Autodesk Fusion 360 part; units mm, degrees
(part 4 of 5)
sketch "Sketch5" plane through (0, 0, 10) normal (0, 0, 1) x (-1, 0, 0)
  arc A0 (206.7946, 25.828) -> (204.1076, 15.8) centre (264.6494, 4.9519) ccw
  arc A1 (201.8483, 14.174) -> (204.1076, 15.8) centre (202.1389, 16.1527) ccw
  line L0 (201.8483, 14.174) -> (193.8046, 15.3551)
  spline S0 degree 5 poles (193.8046, 15.3551) (193.7529, 15.3627) (193.6493, 15.3762) (193.4936, 15.3914) (193.2854, 15.4021) (193.0241, 15.4024) (192.7621, 15.3935) (192.4998, 15.379) (192.2373, 15.3616) (191.9747, 15.342) (191.712, 15.3201) (191.4492, 15.2951) (191.1864, 15.266) (190.9235, 15.2323) (190.6604, 15.1939) (190.3974, 15.1514) (190.1343, 15.1054) (189.8714, 15.0564) (189.6085, 15.0048) (189.3457, 14.9507) (189.083, 14.8941) (188.8205, 14.8347) (188.5581, 14.7725) (188.2959, 14.7074) (188.0338, 14.6394) (187.7718, 14.5688) (187.5101, 14.4956) (187.2485, 14.42) (186.9872, 14.342) (186.7261, 14.2617) (186.4653, 14.1791) (186.2047, 14.0941) (185.9443, 14.0069) (185.6842, 13.9173) (185.4244, 13.8255) (185.1649, 13.7314) (184.9057, 13.6352) (184.6467, 13.5369) (184.3881, 13.4364) (184.1298, 13.3338) (183.8719, 13.2292) (183.6143, 13.1226) (183.357, 13.0139) (183.1001, 12.9031) (182.8435, 12.7904) (182.5874, 12.6758) (182.3316, 12.5591) (182.0762, 12.4406) (181.8212, 12.3201) (181.5665, 12.1977) (181.3123, 12.0735) (181.0585, 11.9474) (180.8052, 11.8194) (180.5522, 11.6897) (180.2997, 11.5581) (180.0477, 11.4246) (179.7961, 11.2895) (179.5449, 11.1525) (179.2942, 11.0138) (179.044, 10.8733) (178.7943, 10.7311) (178.545, 10.5872) (178.2962, 10.4415) (178.048, 10.2942) (177.8002, 10.1451) (177.5529, 9.9945) (177.3062, 9.8421) (177.0599, 9.6881) (176.8142, 9.5325) (176.5691, 9.3752) (176.3244, 9.2163) (176.1291, 9.0879) (175.9829, 8.9909) (175.8855, 8.9259) (175.8369, 8.8933) knots 0 0 0 0 0 0 0.01428571 0.02857143 0.04285714 0.05714286 0.07142857 0.08571429 0.1 0.11428571 0.12857143 0.14285714 0.15714286 0.17142857 0.18571429 0.2 0.21428571 0.22857143 0.24285714 0.25714286 0.27142857 0.28571429 0.3 0.31428571 0.32857143 0.34285714 0.35714286 0.37142857 0.38571429 0.4 0.41428571 0.42857143 0.44285714 0.45714286 0.47142857 0.48571429 0.5 0.51428571 0.52857143 0.54285714 0.55714286 0.57142857 0.58571429 0.6 0.61428571 0.62857143 0.64285714 0.65714286 0.67142857 0.68571429 0.7 0.71428571 0.72857143 0.74285714 0.75714286 0.77142857 0.78571429 0.8 0.81428571 0.82857143 0.84285714 0.85714286 0.87142857 0.88571429 0.9 0.91428571 0.92857143 0.94285714 0.95714286 0.97142857 0.98571429 1 1 1 1 1 1
  arc A2 (175.8369, 8.8933) -> (175.8369, 1.0104) centre (264.6494, 4.9519) ccw
  spline S1 degree 5 poles (175.8369, 1.0104) (175.8855, 0.9779) (175.9829, 0.9129) (176.1291, 0.8158) (176.3244, 0.6874) (176.5691, 0.5285) (176.8142, 0.3713) (177.0599, 0.2156) (177.3062, 0.0616) (177.5529, -0.0907) (177.8002, -0.2414) (178.048, -0.3905) (178.2962, -0.5378) (178.545, -0.6834) (178.7943, -0.8274) (179.044, -0.9696) (179.2942, -1.11) (179.5449, -1.2488) (179.7961, -1.3857) (180.0477, -1.5209) (180.2997, -1.6543) (180.5522, -1.7859) (180.8052, -1.9157) (181.0585, -2.0437) (181.3123, -2.1698) (181.5665, -2.294) (181.8212, -2.4164) (182.0762, -2.5368) (182.3316, -2.6554) (182.5874, -2.772) (182.8435, -2.8867) (183.1001, -2.9994) (183.357, -3.1101) (183.6143, -3.2188) (183.8719, -3.3255) (184.1298, -3.4301) (184.3881, -3.5327) (184.6467, -3.6331) (184.9057, -3.7315) (185.1649, -3.8277) (185.4244, -3.9218) (185.6842, -4.0136) (185.9443, -4.1031) (186.2047, -4.1904) (186.4653, -4.2753) (186.7261, -4.358) (186.9872, -4.4383) (187.2485, -4.5163) (187.5101, -4.5919) (187.7718, -4.6651) (188.0338, -4.7357) (188.2959, -4.8036) (188.5581, -4.8688) (188.8205, -4.931) (189.083, -4.9903) (189.3457, -5.047) (189.6085, -5.1011) (189.8714, -5.1527) (190.1343, -5.2017) (190.3974, -5.2477) (190.6604, -5.2902) (190.9235, -5.3286) (191.1864, -5.3623) (191.4492, -5.3914) (191.712, -5.4164) (191.9747, -5.4383) (192.2373, -5.4578) (192.4998, -5.4753) (192.7621, -5.4898) (193.0241, -5.4987) (193.2854, -5.4984) (193.4936, -5.4877) (193.6493, -5.4725) (193.7529, -5.459) (193.8046, -5.4514) knots -1 -1 -1 -1 -1 -1 -0.98571429 -0.97142857 -0.95714286 -0.94285714 -0.92857143 -0.91428571 -0.9 -0.88571429 -0.87142857 -0.85714286 -0.84285714 -0.82857143 -0.81428571 -0.8 -0.78571429 -0.77142857 -0.75714286 -0.74285714 -0.72857143 -0.71428571 -0.7 -0.68571429 -0.67142857 -0.65714286 -0.64285714 -0.62857143 -0.61428571 -0.6 -0.58571429 -0.57142857 -0.55714286 -0.54285714 -0.52857143 -0.51428571 -0.5 -0.48571429 -0.47142857 -0.45714286 -0.44285714 -0.42857143 -0.41428571 -0.4 -0.38571429 -0.37142857 -0.35714286 -0.34285714 -0.32857143 -0.31428571 -0.3 -0.28571429 -0.27142857 -0.25714286 -0.24285714 -0.22857143 -0.21428571 -0.2 -0.18571429 -0.17142857 -0.15714286 -0.14285714 -0.12857143 -0.11428571 -0.1 -0.08571429 -0.07142857 -0.05714286 -0.04285714 -0.02857143 -0.01428571 0 0 0 0 0 0
  line L1 (193.8046, -5.4514) -> (201.8483, -4.2702)
  arc A3 (204.1076, -5.8963) -> (201.8483, -4.2702) centre (202.1389, -6.249) ccw
  arc A4 (204.1076, -5.8963) -> (206.7946, -15.9243) centre (264.6494, 4.9519) ccw
  arc A5 (205.651, -18.4621) -> (206.7946, -15.9243) centre (204.9133, -16.6032) ccw
  line L2 (205.651, -18.4621) -> (198.0944, -21.461)
  spline S2 degree 5 poles (198.0944, -21.461) (198.0458, -21.4803) (197.9494, -21.5204) (197.8069, -21.5851) (197.6212, -21.68) (197.3948, -21.8104) (197.1724, -21.9491) (196.9524, -22.0928) (196.7338, -22.2391) (196.5162, -22.3874) (196.2996, -22.5377) (196.0846, -22.6907) (195.8715, -22.8473) (195.6607, -23.008) (195.452, -23.1727) (195.2455, -23.3411) (195.0407, -23.5125) (194.8375, -23.6864) (194.6356, -23.8625) (194.4351, -24.0407) (194.2359, -24.2211) (194.0383, -24.4038) (193.8421, -24.5889) (193.6475, -24.7764) (193.4545, -24.9663) (193.263, -25.1584) (193.0729, -25.3527) (192.8842, -25.549) (192.6969, -25.7472) (192.511, -25.9473) (192.3264, -26.1492) (192.1431, -26.3531) (191.9613, -26.5588) (191.7808, -26.7664) (191.6017, -26.9759) (191.424, -27.1871) (191.2476, -27.4) (191.0726, -27.6147) (190.8988, -27.831) (190.7264, -28.0489) (190.5553, -28.2685) (190.3856, -28.4897) (190.2171, -28.7125) (190.05, -28.9368) (189.8842, -29.1627) (189.7197, -29.3901) (189.5564, -29.619) (189.3945, -29.8494) (189.2339, -30.0812) (189.0746, -30.3145) (188.9166, -30.5492) (188.7598, -30.7853) (188.6044, -31.0228) (188.4502, -31.2616) (188.2974, -31.5019) (188.1458, -31.7434) (187.9955, -31.9863) (187.8465, -32.2305) (187.6987, -32.476) (187.5523, -32.7227) (187.4071, -32.9708) (187.2632, -33.22) (187.1206, -33.4706) (186.9792, -33.7223) (186.8391, -33.9752) (186.7003, -34.2294) (186.5628, -34.4847) (186.4266, -34.7412) (186.2916, -34.9988) (186.1579, -35.2576) (186.0255, -35.5175) (185.9206, -35.7264) (185.8425, -35.8835) (185.7906, -35.9885) (185.7648, -36.0411) knots 0 0 0 0 0 0 0.01428571 0.02857143 0.04285714 0.05714286 0.07142857 0.08571429 0.1 0.11428571 0.12857143 0.14285714 0.15714286 0.17142857 0.18571429 0.2 0.21428571 0.22857143 0.24285714 0.25714286 0.27142857 0.28571429 0.3 0.31428571 0.32857143 0.34285714 0.35714286 0.37142857 0.38571429 0.4 0.41428571 0.42857143 0.44285714 0.45714286 0.47142857 0.48571429 0.5 0.51428571 0.52857143 0.54285714 0.55714286 0.57142857 0.58571429 0.6 0.61428571 0.62857143 0.64285714 0.65714286 0.67142857 0.68571429 0.7 0.71428571 0.72857143 0.74285714 0.75714286 0.77142857 0.78571429 0.8 0.81428571 0.82857143 0.84285714 0.85714286 0.87142857 0.88571429 0.9 0.91428571 0.92857143 0.94285714 0.95714286 0.97142857 0.98571429 1 1 1 1 1 1
  arc A6 (185.7648, -36.0411) -> (189.7062, -42.8678) centre (264.6494, 4.9519) ccw
  spline S3 degree 5 poles (189.7062, -42.8678) (189.7646, -42.8717) (189.8815, -42.8793) (190.0566, -42.8902) (190.2899, -42.9038) (190.5813, -42.9191) (190.8722, -42.9327) (191.1628, -42.9446) (191.4531, -42.9548) (191.7429, -42.9634) (192.0324, -42.9703) (192.3215, -42.9755) (192.6102, -42.9789) (192.8985, -42.9807) (193.1863, -42.9807) (193.4737, -42.979) (193.7606, -42.9755) (194.0471, -42.9703) (194.3331, -42.9633) (194.6186, -42.9546) (194.9035, -42.9441) (195.188, -42.9318) (195.472, -42.9178) (195.7554, -42.9019) (196.0382, -42.8842) (196.3205, -42.8647) (196.6022, -42.8434) (196.8832, -42.8202) (197.1637, -42.7952) (197.4436, -42.7683) (197.7227, -42.7395) (198.0013, -42.7088) (198.2791, -42.6763) (198.5563, -42.6418) (198.8327, -42.6053) (199.1084, -42.5669) (199.3834, -42.5266) (199.6576, -42.4843) (199.931, -42.44) (200.2036, -42.3938) (200.4754, -42.3454) (200.7463, -42.2951) (201.0163, -42.2426) (201.2854, -42.188) (201.5536, -42.1312) (201.8208, -42.0723) (202.087, -42.0113) (202.3523, -41.9482) (202.6167, -41.8829) (202.8799, -41.8155) (203.1421, -41.7457) (203.4031, -41.6734) (203.6627, -41.5987) (203.9211, -41.5214) (204.1781, -41.4415) (204.4339, -41.3593) (204.6885, -41.2747) (204.942, -41.188) (205.1942, -41.0989) (205.4451, -41.0073) (205.6941, -40.9125) (205.9411, -40.8142) (206.1857, -40.712) (206.4278, -40.6058) (206.6679, -40.4961) (206.9063, -40.3837) (207.1435, -40.2693) (207.3796, -40.1531) (207.614, -40.0345) (207.8453, -39.9113) (208.0715, -39.7804) (208.2465, -39.667) (208.3737, -39.576) (208.4567, -39.5125) (208.4977, -39.4801) knots -1 -1 -1 -1 -1 -1 -0.98571429 -0.97142857 -0.95714286 -0.94285714 -0.92857143 -0.91428571 -0.9 -0.88571429 -0.87142857 -0.85714286 -0.84285714 -0.82857143 -0.81428571 -0.8 -0.78571429 -0.77142857 -0.75714286 -0.74285714 -0.72857143 -0.71428571 -0.7 -0.68571429 -0.67142857 -0.65714286 -0.64285714 -0.62857143 -0.61428571 -0.6 -0.58571429 -0.57142857 -0.55714286 -0.54285714 -0.52857143 -0.51428571 -0.5 -0.48571429 -0.47142857 -0.45714286 -0.44285714 -0.42857143 -0.41428571 -0.4 -0.38571429 -0.37142857 -0.35714286 -0.34285714 -0.32857143 -0.31428571 -0.3 -0.28571429 -0.27142857 -0.25714286 -0.24285714 -0.22857143 -0.21428571 -0.2 -0.18571429 -0.17142857 -0.15714286 -0.14285714 -0.12857143 -0.11428571 -0.1 -0.08571429 -0.07142857 -0.05714286 -0.04285714 -0.02857143 -0.01428571 0 0 0 0 0 0
  line L3 (208.4977, -39.4801) -> (214.8731, -34.4353)
  arc A7 (217.6427, -34.7138) -> (214.8731, -34.4353) centre (216.1142, -36.0036) ccw
  arc A8 (217.6427, -34.7138) -> (224.9837, -42.0549) centre (264.6494, 4.9519) ccw
  arc A9 (225.2623, -44.8244) -> (224.9837, -42.0549) centre (223.6939, -43.5834) ccw
  line L4 (225.2623, -44.8244) -> (220.2175, -51.1999)
  spline S4 degree 5 poles (220.2175, -51.1999) (220.1851, -51.2409) (220.1216, -51.3238) (220.0306, -51.4511) (219.9172, -51.6261) (219.7863, -51.8522) (219.6631, -52.0835) (219.5444, -52.318) (219.4283, -52.554) (219.3139, -52.7913) (219.2015, -53.0297) (219.0918, -53.2697) (218.9856, -53.5119) (218.8833, -53.7565) (218.785, -54.0035) (218.6903, -54.2525) (218.5987, -54.5033) (218.5096, -54.7556) (218.4228, -55.009) (218.3383, -55.2637) (218.256, -55.5195) (218.1762, -55.7765) (218.0989, -56.0348) (218.0241, -56.2945) (217.9519, -56.5555) (217.8821, -56.8176) (217.8146, -57.0809) (217.7494, -57.3452) (217.6862, -57.6105) (217.6252, -57.8768) (217.5664, -58.144) (217.5096, -58.4122) (217.455, -58.6813) (217.4025, -58.9513) (217.3521, -59.2222) (217.3038, -59.494) (217.2575, -59.7666) (217.2133, -60.04) (217.171, -60.3142) (217.1306, -60.5892) (217.0923, -60.8649) (217.0558, -61.1413) (217.0213, -61.4184) (216.9887, -61.6963) (216.9581, -61.9748) (216.9293, -62.254) (216.9024, -62.5339) (216.8774, -62.8143) (216.8542, -63.0954) (216.8329, -63.3771) (216.8134, -63.6594) (216.7957, -63.9422) (216.7798, -64.2256) (216.7657, -64.5096) (216.7535, -64.794) (216.743, -65.079) (216.7342, -65.3645) (216.7273, -65.6505) (216.7221, -65.937) (216.7186, -66.2239) (216.7169, -66.5113) (216.7169, -66.7991) (216.7187, -67.0874) (216.7221, -67.3761) (216.7273, -67.6652) (216.7342, -67.9546) (216.7427, -68.2445) (216.753, -68.5348) (216.7649, -68.8254) (216.7785, -69.1163) (216.7938, -69.4076) (216.8074, -69.641) (216.8183, -69.8161) (216.8259, -69.933) (216.8298, -69.9914) knots 0 0 0 0 0 0 0.01428571 0.02857143 0.04285714 0.05714286 0.07142857 0.08571429 0.1 0.11428571 0.12857143 0.14285714 0.15714286 0.17142857 0.18571429 0.2 0.21428571 0.22857143 0.24285714 0.25714286 0.27142857 0.28571429 0.3 0.31428571 0.32857143 0.34285714 0.35714286 0.37142857 0.38571429 0.4 0.41428571 0.42857143 0.44285714 0.45714286 0.47142857 0.48571429 0.5 0.51428571 0.52857143 0.54285714 0.55714286 0.57142857 0.58571429 0.6 0.61428571 0.62857143 0.64285714 0.65714286 0.67142857 0.68571429 0.7 0.71428571 0.72857143 0.74285714 0.75714286 0.77142857 0.78571429 0.8 0.81428571 0.82857143 0.84285714 0.85714286 0.87142857 0.88571429 0.9 0.91428571 0.92857143 0.94285714 0.95714286 0.97142857 0.98571429 1 1 1 1 1 1
  arc A10 (216.8298, -69.9914) -> (223.6565, -73.9328) centre (264.6494, 4.9519) ccw
  spline S5 degree 5 poles (223.6565, -73.9328) (223.7091, -73.9069) (223.814, -73.8551) (223.9712, -73.777) (224.18, -73.6721) (224.44, -73.5397) (224.6987, -73.406) (224.9564, -73.271) (225.2129, -73.1348) (225.4682, -72.9972) (225.7223, -72.8584) (225.9753, -72.7184) (226.227, -72.577) (226.4775, -72.4344) (226.7268, -72.2905) (226.9748, -72.1453) (227.2216, -71.9989) (227.4671, -71.8511) (227.7113, -71.7021) (227.9542, -71.5518) (228.1957, -71.4002) (228.4359, -71.2473) (228.6748, -71.0932) (228.9123, -70.9377) (229.1484, -70.781) (229.3831, -70.623) (229.6164, -70.4637) (229.8482, -70.303) (230.0786, -70.1411) (230.3075, -69.9779) (230.5349, -69.8134) (230.7608, -69.6476) (230.9851, -69.4804) (231.2079, -69.312) (231.4291, -69.1422) (231.6486, -68.9711) (231.8666, -68.7987) (232.0829, -68.625) (232.2976, -68.45) (232.5105, -68.2736) (232.7217, -68.0958) (232.9311, -67.9167) (233.1387, -67.7363) (233.3445, -67.5544) (233.5483, -67.3712) (233.7503, -67.1866) (233.9504, -67.0007) (234.1486, -66.8133) (234.3449, -66.6247) (234.5391, -66.4346) (234.7313, -66.2431) (234.9212, -66.05) (235.1087, -65.8555) (235.2938, -65.6593) (235.4764, -65.4617) (235.6568, -65.2625) (235.8351, -65.062) (236.0112, -64.8601) (236.1851, -64.6569) (236.3565, -64.4521) (236.5248, -64.2455) (236.6895, -64.0369) (236.8503, -63.8261) (237.0069, -63.613) (237.1599, -63.398) (237.3102, -63.1814) (237.4584, -62.9638) (237.6048, -62.7451) (237.7485, -62.5252) (237.8872, -62.3028) (238.0176, -62.0764) (238.1125, -61.8907) (238.1772, -61.7482) (238.2173, -61.6518) (238.2365, -61.6032) knots -1 -1 -1 -1 -1 -1 -0.98571429 -0.97142857 -0.95714286 -0.94285714 -0.92857143 -0.91428571 -0.9 -0.88571429 -0.87142857 -0.85714286 -0.84285714 -0.82857143 -0.81428571 -0.8 -0.78571429 -0.77142857 -0.75714286 -0.74285714 -0.72857143 -0.71428571 -0.7 -0.68571429 -0.67142857 -0.65714286 -0.64285714 -0.62857143 -0.61428571 -0.6 -0.58571429 -0.57142857 -0.55714286 -0.54285714 -0.52857143 -0.51428571 -0.5 -0.48571429 -0.47142857 -0.45714286 -0.44285714 -0.42857143 -0.41428571 -0.4 -0.38571429 -0.37142857 -0.35714286 -0.34285714 -0.32857143 -0.31428571 -0.3 -0.28571429 -0.27142857 -0.25714286 -0.24285714 -0.22857143 -0.21428571 -0.2 -0.18571429 -0.17142857 -0.15714286 -0.14285714 -0.12857143 -0.11428571 -0.1 -0.08571429 -0.07142857 -0.05714286 -0.04285714 -0.02857143 -0.01428571 0 0 0 0 0 0
  line L5 (238.2365, -61.6032) -> (241.2355, -54.0465)
  arc A11 (243.7733, -52.903) -> (241.2355, -54.0465) centre (243.0944, -54.7843) ccw
  arc A12 (243.7733, -52.903) -> (253.8013, -55.59) centre (264.6494, 4.9519) ccw
  arc A13 (255.4273, -57.8492) -> (253.8013, -55.59) centre (253.4486, -57.5587) ccw
  line L6 (255.4273, -57.8492) -> (254.2461, -65.8929)
  spline S6 degree 5 poles (254.2461, -65.8929) (254.2386, -65.9447) (254.225, -66.0482) (254.2099, -66.2039) (254.1992, -66.4122) (254.1989, -66.6735) (254.2078, -66.9354) (254.2223, -67.1978) (254.2397, -67.4603) (254.2593, -67.7229) (254.2812, -67.9856) (254.3062, -68.2483) (254.3353, -68.5112) (254.369, -68.7741) (254.4074, -69.0371) (254.4499, -69.3002) (254.4959, -69.5632) (254.5449, -69.8262) (254.5965, -70.0891) (254.6506, -70.3519) (254.7072, -70.6145) (254.7666, -70.8771) (254.8288, -71.1395) (254.8939, -71.4017) (254.9619, -71.6638) (255.0325, -71.9258) (255.1057, -72.1875) (255.1813, -72.449) (255.2593, -72.7104) (255.3396, -72.9715) (255.4222, -73.2323) (255.5072, -73.4929) (255.5944, -73.7533) (255.684, -74.0134) (255.7758, -74.2732) (255.8699, -74.5327) (255.9661, -74.7919) (256.0644, -75.0508) (256.1649, -75.3095) (256.2675, -75.5677) (256.3721, -75.8257) (256.4787, -76.0833) (256.5874, -76.3406) (256.6981, -76.5975) (256.8109, -76.854) (256.9255, -77.1102) (257.0422, -77.366) (257.1607, -77.6214) (257.2812, -77.8764) (257.4036, -78.131) (257.5278, -78.3852) (257.6539, -78.639) (257.7819, -78.8924) (257.9116, -79.1453) (258.0432, -79.3978) (258.1766, -79.6499) (258.3118, -79.9015) (258.4488, -80.1527) (258.5875, -80.4033) (258.728, -80.6536) (258.8702, -80.9033) (259.0141, -81.1526) (259.1598, -81.4013) (259.3071, -81.6496) (259.4561, -81.8974) (259.6068, -82.1447) (259.7592, -82.3914) (259.9132, -82.6376) (260.0688, -82.8834) (260.2261, -83.1285) (260.385, -83.3732) (260.5134, -83.5685) (260.6104, -83.7147) (260.6754, -83.8121) (260.708, -83.8607) knots 0 0 0 0 0 0 0.01428571 0.02857143 0.04285714 0.05714286 0.07142857 0.08571429 0.1 0.11428571 0.12857143 0.14285714 0.15714286 0.17142857 0.18571429 0.2 0.21428571 0.22857143 0.24285714 0.25714286 0.27142857 0.28571429 0.3 0.31428571 0.32857143 0.34285714 0.35714286 0.37142857 0.38571429 0.4 0.41428571 0.42857143 0.44285714 0.45714286 0.47142857 0.48571429 0.5 0.51428571 0.52857143 0.54285714 0.55714286 0.57142857 0.58571429 0.6 0.61428571 0.62857143 0.64285714 0.65714286 0.67142857 0.68571429 0.7 0.71428571 0.72857143 0.74285714 0.75714286 0.77142857 0.78571429 0.8 0.81428571 0.82857143 0.84285714 0.85714286 0.87142857 0.88571429 0.9 0.91428571 0.92857143 0.94285714 0.95714286 0.97142857 0.98571429 1 1 1 1 1 1
  arc A14 (260.708, -83.8607) -> (268.5908, -83.8607) centre (264.6494, 4.9519) ccw
  spline S7 degree 5 poles (268.5908, -83.8607) (268.6234, -83.8121) (268.6884, -83.7147) (268.7855, -83.5685) (268.9139, -83.3732) (269.0728, -83.1285) (269.23, -82.8834) (269.3857, -82.6376) (269.5397, -82.3914) (269.692, -82.1447) (269.8427, -81.8974) (269.9917, -81.6496) (270.1391, -81.4013) (270.2847, -81.1526) (270.4287, -80.9033) (270.5709, -80.6536) (270.7113, -80.4033) (270.8501, -80.1527) (270.987, -79.9015) (271.1222, -79.6499) (271.2556, -79.3978) (271.3872, -79.1453) (271.517, -78.8924) (271.645, -78.639) (271.7711, -78.3852) (271.8953, -78.131) (272.0177, -77.8764) (272.1381, -77.6214) (272.2567, -77.366) (272.3733, -77.1102) (272.488, -76.854) (272.6007, -76.5975) (272.7114, -76.3406) (272.8201, -76.0833) (272.9268, -75.8257) (273.0314, -75.5677) (273.134, -75.3095) (273.2344, -75.0508) (273.3328, -74.7919) (273.429, -74.5327) (273.5231, -74.2732) (273.6149, -74.0134) (273.7044, -73.7533) (273.7917, -73.4929) (273.8766, -73.2323) (273.9592, -72.9715) (274.0396, -72.7104) (274.1175, -72.449) (274.1932, -72.1875) (274.2664, -71.9258) (274.337, -71.6638) (274.4049, -71.4017) (274.47, -71.1395) (274.5323, -70.8771) (274.5916, -70.6145) (274.6483, -70.3519) (274.7024, -70.0891) (274.754, -69.8262) (274.803, -69.5632) (274.849, -69.3002) (274.8915, -69.0371) (274.9299, -68.7741) (274.9636, -68.5112) (274.9927, -68.2483) (275.0177, -67.9856) (275.0396, -67.7229) (275.0591, -67.4603) (275.0766, -67.1978) (275.0911, -66.9354) (275.1, -66.6735) (275.0997, -66.4122) (275.089, -66.2039) (275.0738, -66.0482) (275.0603, -65.9447) (275.0527, -65.8929) knots -1 -1 -1 -1 -1 -1 -0.98571429 -0.97142857 -0.95714286 -0.94285714 -0.92857143 -0.91428571 -0.9 -0.88571429 -0.87142857 -0.85714286 -0.84285714 -0.82857143 -0.81428571 -0.8 -0.78571429 -0.77142857 -0.75714286 -0.74285714 -0.72857143 -0.71428571 -0.7 -0.68571429 -0.67142857 -0.65714286 -0.64285714 -0.62857143 -0.61428571 -0.6 -0.58571429 -0.57142857 -0.55714286 -0.54285714 -0.52857143 -0.51428571 -0.5 -0.48571429 -0.47142857 -0.45714286 -0.44285714 -0.42857143 -0.41428571 -0.4 -0.38571429 -0.37142857 -0.35714286 -0.34285714 -0.32857143 -0.31428571 -0.3 -0.28571429 -0.27142857 -0.25714286 -0.24285714 -0.22857143 -0.21428571 -0.2 -0.18571429 -0.17142857 -0.15714286 -0.14285714 -0.12857143 -0.11428571 -0.1 -0.08571429 -0.07142857 -0.05714286 -0.04285714 -0.02857143 -0.01428571 0 0 0 0 0 0
  line L7 (275.0527, -65.8929) -> (273.8715, -57.8492)
  arc A15 (275.4976, -55.59) -> (273.8715, -57.8492) centre (275.8503, -57.5587) ccw
  arc A16 (275.4976, -55.59) -> (285.5256, -52.903) centre (264.6494, 4.9519) ccw
  arc A17 (288.0634, -54.0465) -> (285.5256, -52.903) centre (286.2045, -54.7843) ccw
  line L8 (288.0634, -54.0465) -> (291.0623, -61.6032)
  spline S8 degree 5 poles (291.0623, -61.6032) (291.0816, -61.6518) (291.1217, -61.7482) (291.1864, -61.8907) (291.2813, -62.0764) (291.4117, -62.3028) (291.5503, -62.5252) (291.6941, -62.7451) (291.8404, -62.9638) (291.9887, -63.1814) (292.139, -63.398) (292.292, -63.613) (292.4486, -63.8261) (292.6093, -64.0369) (292.774, -64.2455) (292.9424, -64.4521) (293.1138, -64.6569) (293.2877, -64.8601) (293.4638, -65.062) (293.642, -65.2625) (293.8224, -65.4617) (294.0051, -65.6593) (294.1902, -65.8555) (294.3777, -66.05) (294.5676, -66.2431) (294.7597, -66.4346) (294.954, -66.6247) (295.1503, -66.8133) (295.3485, -67.0007) (295.5486, -67.1866) (295.7505, -67.3712) (295.9544, -67.5544) (296.1601, -67.7363) (296.3677, -67.9167) (296.5772, -68.0958) (296.7884, -68.2736) (297.0013, -68.45) (297.216, -68.625) (297.4323, -68.7987) (297.6502, -68.9711) (297.8698, -69.1422) (298.091, -69.312) (298.3138, -69.4804) (298.5381, -69.6476) (298.764, -69.8134) (298.9914, -69.9779) (299.2203, -70.1411) (299.4507, -70.303) (299.6825, -70.4637) (299.9158, -70.623) (300.1505, -70.781) (300.3866, -70.9377) (300.6241, -71.0932) (300.8629, -71.2473) (301.1032, -71.4002) (301.3447, -71.5518) (301.5876, -71.7021) (301.8318, -71.8511) (302.0773, -71.9989) (302.324, -72.1453) (302.5721, -72.2905) (302.8213, -72.4344) (303.0719, -72.577) (303.3236, -72.7184) (303.5765, -72.8584) (303.8307, -72.9972) (304.086, -73.1348) (304.3425, -73.271) (304.6001, -73.406) (304.8589, -73.5397) (305.1188, -73.6721) (305.3277, -73.777) (305.4848, -73.8551) (305.5898, -73.9069) (305.6424, -73.9328) knots 0 0 0 0 0 0 0.01428571 0.02857143 0.04285714 0.05714286 0.07142857 0.08571429 0.1 0.11428571 0.12857143 0.14285714 0.15714286 0.17142857 0.18571429 0.2 0.21428571 0.22857143 0.24285714 0.25714286 0.27142857 0.28571429 0.3 0.31428571 0.32857143 0.34285714 0.35714286 0.37142857 0.38571429 0.4 0.41428571 0.42857143 0.44285714 0.45714286 0.47142857 0.48571429 0.5 0.51428571 0.52857143 0.54285714 0.55714286 0.57142857 0.58571429 0.6 0.61428571 0.62857143 0.64285714 0.65714286 0.67142857 0.68571429 0.7 0.71428571 0.72857143 0.74285714 0.75714286 0.77142857 0.78571429 0.8 0.81428571 0.82857143 0.84285714 0.85714286 0.87142857 0.88571429 0.9 0.91428571 0.92857143 0.94285714 0.95714286 0.97142857 0.98571429 1 1 1 1 1 1
  arc A18 (305.6424, -73.9328) -> (312.4691, -69.9914) centre (264.6494, 4.9519) ccw
  spline S9 degree 5 poles (312.4691, -69.9914) (312.473, -69.933) (312.4806, -69.8161) (312.4915, -69.641) (312.5051, -69.4076) (312.5203, -69.1163) (312.534, -68.8254) (312.5459, -68.5348) (312.5561, -68.2445) (312.5647, -67.9546) (312.5716, -67.6652) (312.5768, -67.3761) (312.5802, -67.0874) (312.582, -66.7991) (312.582, -66.5113) (312.5803, -66.2239) (312.5768, -65.937) (312.5716, -65.6505) (312.5646, -65.3645) (312.5559, -65.079) (312.5454, -64.794) (312.5331, -64.5096) (312.5191, -64.2256) (312.5032, -63.9422) (312.4855, -63.6594) (312.466, -63.3771) (312.4447, -63.0954) (312.4215, -62.8143) (312.3965, -62.5339) (312.3696, -62.254) (312.3408, -61.9748) (312.3101, -61.6963) (312.2775, -61.4184) (312.243, -61.1413) (312.2066, -60.8649) (312.1682, -60.5892) (312.1279, -60.3142) (312.0856, -60.04) (312.0413, -59.7666) (311.9951, -59.494) (311.9467, -59.2222) (311.8964, -58.9513) (311.8439, -58.6813) (311.7893, -58.4122) (311.7325, -58.144) (311.6736, -57.8768) (311.6126, -57.6105) (311.5495, -57.3452) (311.4842, -57.0809) (311.4168, -56.8176) (311.347, -56.5555) (311.2747, -56.2945) (311.2, -56.0348) (311.1227, -55.7765) (311.0428, -55.5195) (310.9606, -55.2637) (310.876, -55.009) (310.7893, -54.7556) (310.7002, -54.5033) (310.6086, -54.2525) (310.5138, -54.0035) (310.4155, -53.7565) (310.3133, -53.5119) (310.2071, -53.2697) (310.0974, -53.0297) (309.985, -52.7913) (309.8706, -52.554) (309.7544, -52.318) (309.6358, -52.0835) (309.5126, -51.8522) (309.3817, -51.6261) (309.2683, -51.4511) (309.1773, -51.3238) (309.1138, -51.2409) (309.0814, -51.1999) knots -1 -1 -1 -1 -1 -1 -0.98571429 -0.97142857 -0.95714286 -0.94285714 -0.92857143 -0.91428571 -0.9 -0.88571429 -0.87142857 -0.85714286 -0.84285714 -0.82857143 -0.81428571 -0.8 -0.78571429 -0.77142857 -0.75714286 -0.74285714 -0.72857143 -0.71428571 -0.7 -0.68571429 -0.67142857 -0.65714286 -0.64285714 -0.62857143 -0.61428571 -0.6 -0.58571429 -0.57142857 -0.55714286 -0.54285714 -0.52857143 -0.51428571 -0.5 -0.48571429 -0.47142857 -0.45714286 -0.44285714 -0.42857143 -0.41428571 -0.4 -0.38571429 -0.37142857 -0.35714286 -0.34285714 -0.32857143 -0.31428571 -0.3 -0.28571429 -0.27142857 -0.25714286 -0.24285714 -0.22857143 -0.21428571 -0.2 -0.18571429 -0.17142857 -0.15714286 -0.14285714 -0.12857143 -0.11428571 -0.1 -0.08571429 -0.07142857 -0.05714286 -0.04285714 -0.02857143 -0.01428571 0 0 0 0 0 0
  line L9 (309.0814, -51.1999) -> (304.0366, -44.8244)
  arc A19 (304.3151, -42.0549) -> (304.0366, -44.8244) centre (305.6049, -43.5834) ccw
  arc A20 (304.3151, -42.0549) -> (311.6562, -34.7138) centre (264.6494, 4.9519) ccw
  arc A21 (314.4257, -34.4353) -> (311.6562, -34.7138) centre (313.1847, -36.0036) ccw
  line L10 (314.4257, -34.4353) -> (320.8012, -39.4801)
  spline S10 degree 5 poles (320.8012, -39.4801) (320.8422, -39.5125) (320.9251, -39.576) (321.0524, -39.667) (321.2274, -39.7804) (321.4535, -39.9113) (321.6848, -40.0345) (321.9193, -40.1531) (322.1553, -40.2693) (322.3926, -40.3837) (322.631, -40.4961) (322.871, -40.6058) (323.1132, -40.712) (323.3578, -40.8142) (323.6048, -40.9125) (323.8538, -41.0073) (324.1046, -41.0989) (324.3569, -41.188) (324.6103, -41.2747) (324.865, -41.3593) (325.1207, -41.4415) (325.3778, -41.5214) (325.6361, -41.5987) (325.8958, -41.6734) (326.1568, -41.7457) (326.4189, -41.8155) (326.6822, -41.8829) (326.9465, -41.9482) (327.2118, -42.0113) (327.4781, -42.0723) (327.7453, -42.1312) (328.0135, -42.188) (328.2826, -42.2426) (328.5526, -42.2951) (328.8235, -42.3454) (329.0953, -42.3938) (329.3679, -42.44) (329.6413, -42.4843) (329.9155, -42.5266) (330.1905, -42.5669) (330.4662, -42.6053) (330.7426, -42.6418) (331.0197, -42.6763) (331.2976, -42.7088) (331.5761, -42.7395) (331.8553, -42.7683) (332.1352, -42.7952) (332.4156, -42.8202) (332.6967, -42.8434) (332.9784, -42.8647) (333.2607, -42.8842) (333.5435, -42.9019) (333.8269, -42.9178) (334.1108, -42.9318) (334.3953, -42.9441) (334.6803, -42.9546) (334.9658, -42.9633) (335.2518, -42.9703) (335.5383, -42.9755) (335.8252, -42.979) (336.1126, -42.9807) (336.4004, -42.9807) (336.6887, -42.9789) (336.9774, -42.9755) (337.2664, -42.9703) (337.5559, -42.9634) (337.8458, -42.9548) (338.1361, -42.9446) (338.4267, -42.9327) (338.7176, -42.9191) (339.0089, -42.9038) (339.2423, -42.8902) (339.4174, -42.8793) (339.5342, -42.8717) (339.5927, -42.8678) knots 0 0 0 0 0 0 0.01428571 0.02857143 0.04285714 0.05714286 0.07142857 0.08571429 0.1 0.11428571 0.12857143 0.14285714 0.15714286 0.17142857 0.18571429 0.2 0.21428571 0.22857143 0.24285714 0.25714286 0.27142857 0.28571429 0.3 0.31428571 0.32857143 0.34285714 0.35714286 0.37142857 0.38571429 0.4 0.41428571 0.42857143 0.44285714 0.45714286 0.47142857 0.48571429 0.5 0.51428571 0.52857143 0.54285714 0.55714286 0.57142857 0.58571429 0.6 0.61428571 0.62857143 0.64285714 0.65714286 0.67142857 0.68571429 0.7 0.71428571 0.72857143 0.74285714 0.75714286 0.77142857 0.78571429 0.8 0.81428571 0.82857143 0.84285714 0.85714286 0.87142857 0.88571429 0.9 0.91428571 0.92857143 0.94285714 0.95714286 0.97142857 0.98571429 1 1 1 1 1 1
  arc A22 (339.5927, -42.8678) -> (343.5341, -36.0411) centre (264.6494, 4.9519) ccw
  spline S11 degree 5 poles (343.5341, -36.0411) (343.5082, -35.9885) (343.4564, -35.8835) (343.3783, -35.7264) (343.2734, -35.5175) (343.141, -35.2576) (343.0073, -34.9988) (342.8723, -34.7412) (342.7361, -34.4847) (342.5985, -34.2294) (342.4597, -33.9752) (342.3197, -33.7223) (342.1783, -33.4706) (342.0357, -33.22) (341.8918, -32.9708) (341.7466, -32.7227) (341.6002, -32.476) (341.4524, -32.2305) (341.3034, -31.9863) (341.1531, -31.7434) (341.0015, -31.5019) (340.8486, -31.2616) (340.6945, -31.0228) (340.539, -30.7853) (340.3823, -30.5492) (340.2243, -30.3145) (340.065, -30.0812) (339.9043, -29.8494) (339.7424, -29.619) (339.5792, -29.3901) (339.4147, -29.1627) (339.2489, -28.9368) (339.0817, -28.7125) (338.9133, -28.4897) (338.7435, -28.2685) (338.5724, -28.0489) (338.4, -27.831) (338.2263, -27.6147) (338.0513, -27.4) (337.8749, -27.1871) (337.6971, -26.9759) (337.518, -26.7664) (337.3376, -26.5588) (337.1557, -26.3531) (336.9725, -26.1492) (336.7879, -25.9473) (336.602, -25.7472) (336.4146, -25.549) (336.226, -25.3527) (336.0359, -25.1584) (335.8444, -24.9663) (335.6513, -24.7764) (335.4568, -24.5889) (335.2606, -24.4038) (335.0629, -24.2211) (334.8638, -24.0407) (334.6633, -23.8625) (334.4614, -23.6864) (334.2582, -23.5125) (334.0534, -23.3411) (333.8468, -23.1727) (333.6382, -23.008) (333.4274, -22.8473) (333.2143, -22.6907) (332.9993, -22.5377) (332.7827, -22.3874) (332.565, -22.2391) (332.3464, -22.0928) (332.1265, -21.9491) (331.9041, -21.8104) (331.6777, -21.68) (331.492, -21.5851) (331.3495, -21.5204) (331.2531, -21.4803) (331.2045, -21.461) knots -1 -1 -1 -1 -1 -1 -0.98571429 -0.97142857 -0.95714286 -0.94285714 -0.92857143 -0.91428571 -0.9 -0.88571429 -0.87142857 -0.85714286 -0.84285714 -0.82857143 -0.81428571 -0.8 -0.78571429 -0.77142857 -0.75714286 -0.74285714 -0.72857143 -0.71428571 -0.7 -0.68571429 -0.67142857 -0.65714286 -0.64285714 -0.62857143 -0.61428571 -0.6 -0.58571429 -0.57142857 -0.55714286 -0.54285714 -0.52857143 -0.51428571 -0.5 -0.48571429 -0.47142857 -0.45714286 -0.44285714 -0.42857143 -0.41428571 -0.4 -0.38571429 -0.37142857 -0.35714286 -0.34285714 -0.32857143 -0.31428571 -0.3 -0.28571429 -0.27142857 -0.25714286 -0.24285714 -0.22857143 -0.21428571 -0.2 -0.18571429 -0.17142857 -0.15714286 -0.14285714 -0.12857143 -0.11428571 -0.1 -0.08571429 -0.07142857 -0.05714286 -0.04285714 -0.02857143 -0.01428571 0 0 0 0 0 0
  line L11 (331.2045, -21.461) -> (323.6478, -18.4621)
  arc A23 (322.5043, -15.9243) -> (323.6478, -18.4621) centre (324.3856, -16.6032) ccw
  arc A24 (322.5043, -15.9243) -> (325.1913, -5.8963) centre (264.6494, 4.9519) ccw
  arc A25 (327.4505, -4.2702) -> (325.1913, -5.8963) centre (327.16, -6.249) ccw
  line L12 (327.4505, -4.2702) -> (335.4942, -5.4514)
  spline S12 degree 5 poles (335.4942, -5.4514) (335.546, -5.459) (335.6495, -5.4725) (335.8052, -5.4877) (336.0135, -5.4984) (336.2748, -5.4987) (336.5367, -5.4898) (336.7991, -5.4753) (337.0616, -5.4578) (337.3242, -5.4383) (337.5869, -5.4164) (337.8496, -5.3914) (338.1125, -5.3623) (338.3754, -5.3286) (338.6384, -5.2902) (338.9015, -5.2477) (339.1645, -5.2017) (339.4275, -5.1527) (339.6904, -5.1011) (339.9532, -5.047) (340.2158, -4.9903) (340.4784, -4.931) (340.7408, -4.8688) (341.003, -4.8036) (341.2651, -4.7357) (341.5271, -4.6651) (341.7888, -4.5919) (342.0503, -4.5163) (342.3117, -4.4383) (342.5728, -4.358) (342.8336, -4.2753) (343.0942, -4.1904) (343.3546, -4.1031) (343.6147, -4.0136) (343.8745, -3.9218) (344.134, -3.8277) (344.3932, -3.7315) (344.6521, -3.6331) (344.9107, -3.5327) (345.169, -3.4301) (345.427, -3.3255) (345.6846, -3.2188) (345.9419, -3.1101) (346.1988, -2.9994) (346.4553, -2.8867) (346.7115, -2.772) (346.9673, -2.6554) (347.2227, -2.5368) (347.4777, -2.4164) (347.7323, -2.294) (347.9865, -2.1698) (348.2403, -2.0437) (348.4937, -1.9157) (348.7466, -1.7859) (348.9991, -1.6543) (349.2512, -1.5209) (349.5028, -1.3857) (349.7539, -1.2488) (350.0046, -1.11) (350.2548, -0.9696) (350.5046, -0.8274) (350.7539, -0.6834) (351.0026, -0.5378) (351.2509, -0.3905) (351.4987, -0.2414) (351.746, -0.0907) (351.9927, 0.0616) (352.2389, 0.2156) (352.4846, 0.3713) (352.7298, 0.5285) (352.9745, 0.6874) (353.1698, 0.8158) (353.316, 0.9129) (353.4134, 0.9779) (353.462, 1.0104) knots 0 0 0 0 0 0 0.01428571 0.02857143 0.04285714 0.05714286 0.07142857 0.08571429 0.1 0.11428571 0.12857143 0.14285714 0.15714286 0.17142857 0.18571429 0.2 0.21428571 0.22857143 0.24285714 0.25714286 0.27142857 0.28571429 0.3 0.31428571 0.32857143 0.34285714 0.35714286 0.37142857 0.38571429 0.4 0.41428571 0.42857143 0.44285714 0.45714286 0.47142857 0.48571429 0.5 0.51428571 0.52857143 0.54285714 0.55714286 0.57142857 0.58571429 0.6 0.61428571 0.62857143 0.64285714 0.65714286 0.67142857 0.68571429 0.7 0.71428571 0.72857143 0.74285714 0.75714286 0.77142857 0.78571429 0.8 0.81428571 0.82857143 0.84285714 0.85714286 0.87142857 0.88571429 0.9 0.91428571 0.92857143 0.94285714 0.95714286 0.97142857 0.98571429 1 1 1 1 1 1
  arc A26 (353.462, 1.0104) -> (353.462, 8.8933) centre (264.6494, 4.9519) ccw
  spline S13 degree 5 poles (353.462, 8.8933) (353.4134, 8.9259) (353.316, 8.9909) (353.1698, 9.0879) (352.9745, 9.2163) (352.7298, 9.3752) (352.4846, 9.5325) (352.2389, 9.6881) (351.9927, 9.8421) (351.746, 9.9945) (351.4987, 10.1451) (351.2509, 10.2942) (351.0026, 10.4415) (350.7539, 10.5872) (350.5046, 10.7311) (350.2548, 10.8733) (350.0046, 11.0138) (349.7539, 11.1525) (349.5028, 11.2895) (349.2512, 11.4246) (348.9991, 11.5581) (348.7466, 11.6897) (348.4937, 11.8194) (348.2403, 11.9474) (347.9865, 12.0735) (347.7323, 12.1977) (347.4777, 12.3201) (347.2227, 12.4406) (346.9673, 12.5591) (346.7115, 12.6758) (346.4553, 12.7904) (346.1988, 12.9031) (345.9419, 13.0139) (345.6846, 13.1226) (345.427, 13.2292) (345.169, 13.3338) (344.9107, 13.4364) (344.6521, 13.5369) (344.3932, 13.6352) (344.134, 13.7314) (343.8745, 13.8255) (343.6147, 13.9173) (343.3546, 14.0069) (343.0942, 14.0941) (342.8336, 14.1791) (342.5728, 14.2617) (342.3117, 14.342) (342.0503, 14.42) (341.7888, 14.4956) (341.5271, 14.5688) (341.2651, 14.6394) (341.003, 14.7074) (340.7408, 14.7725) (340.4784, 14.8347) (340.2158, 14.8941) (339.9532, 14.9507) (339.6904, 15.0048) (339.4275, 15.0564) (339.1645, 15.1054) (338.9015, 15.1514) (338.6384, 15.1939) (338.3754, 15.2323) (338.1125, 15.266) (337.8496, 15.2951) (337.5869, 15.3201) (337.3242, 15.342) (337.0616, 15.3616) (336.7991, 15.379) (336.5367, 15.3935) (336.2748, 15.4024) (336.0135, 15.4021) (335.8052, 15.3914) (335.6495, 15.3762) (335.546, 15.3627) (335.4942, 15.3551) knots -1 -1 -1 -1 -1 -1 -0.98571429 -0.97142857 -0.95714286 -0.94285714 -0.92857143 -0.91428571 -0.9 -0.88571429 -0.87142857 -0.85714286 -0.84285714 -0.82857143 -0.81428571 -0.8 -0.78571429 -0.77142857 -0.75714286 -0.74285714 -0.72857143 -0.71428571 -0.7 -0.68571429 -0.67142857 -0.65714286 -0.64285714 -0.62857143 -0.61428571 -0.6 -0.58571429 -0.57142857 -0.55714286 -0.54285714 -0.52857143 -0.51428571 -0.5 -0.48571429 -0.47142857 -0.45714286 -0.44285714 -0.42857143 -0.41428571 -0.4 -0.38571429 -0.37142857 -0.35714286 -0.34285714 -0.32857143 -0.31428571 -0.3 -0.28571429 -0.27142857 -0.25714286 -0.24285714 -0.22857143 -0.21428571 -0.2 -0.18571429 -0.17142857 -0.15714286 -0.14285714 -0.12857143 -0.11428571 -0.1 -0.08571429 -0.07142857 -0.05714286 -0.04285714 -0.02857143 -0.01428571 0 0 0 0 0 0
  line L13 (335.4942, 15.3551) -> (327.4505, 14.174)
  arc A27 (325.1913, 15.8) -> (327.4505, 14.174) centre (327.16, 16.1527) ccw
  arc A28 (325.1913, 15.8) -> (322.5043, 25.828) centre (264.6494, 4.9519) ccw
  arc A29 (323.6478, 28.3658) -> (322.5043, 25.828) centre (324.3856, 26.5069) ccw
  line L14 (323.6478, 28.3658) -> (331.2045, 31.3648)
  spline S14 degree 5 poles (331.2045, 31.3648) (331.2531, 31.384) (331.3495, 31.4241) (331.492, 31.4888) (331.6777, 31.5837) (331.9041, 31.7141) (332.1265, 31.8528) (332.3464, 31.9965) (332.565, 32.1429) (332.7827, 32.2911) (332.9993, 32.4414) (333.2143, 32.5944) (333.4274, 32.751) (333.6382, 32.9117) (333.8468, 33.0765) (334.0534, 33.2448) (334.2582, 33.4162) (334.4614, 33.5901) (334.6633, 33.7662) (334.8638, 33.9445) (335.0629, 34.1249) (335.2606, 34.3075) (335.4568, 34.4926) (335.6513, 34.6801) (335.8444, 34.87) (336.0359, 35.0622) (336.226, 35.2564) (336.4146, 35.4527) (336.602, 35.6509) (336.7879, 35.851) (336.9725, 36.053) (337.1557, 36.2568) (337.3376, 36.4626) (337.518, 36.6702) (337.6971, 36.8796) (337.8749, 37.0908) (338.0513, 37.3037) (338.2263, 37.5184) (338.4, 37.7347) (338.5724, 37.9527) (338.7435, 38.1722) (338.9133, 38.3934) (339.0817, 38.6162) (339.2489, 38.8405) (339.4147, 39.0664) (339.5792, 39.2938) (339.7424, 39.5227) (339.9043, 39.7531) (340.065, 39.9849) (340.2243, 40.2182) (340.3823, 40.4529) (340.539, 40.689) (340.6945, 40.9265) (340.8486, 41.1654) (341.0015, 41.4056) (341.1531, 41.6471) (341.3034, 41.89) (341.4524, 42.1342) (341.6002, 42.3797) (341.7466, 42.6265) (341.8918, 42.8745) (342.0357, 43.1238) (342.1783, 43.3743) (342.3197, 43.626) (342.4597, 43.879) (342.5985, 44.1331) (342.7361, 44.3884) (342.8723, 44.6449) (343.0073, 44.9025) (343.141, 45.1613) (343.2734, 45.4213) (343.3783, 45.6301) (343.4564, 45.7872) (343.5082, 45.8922) (343.5341, 45.9448) knots 0 0 0 0 0 0 0.01428571 0.02857143 0.04285714 0.05714286 0.07142857 0.08571429 0.1 0.11428571 0.12857143 0.14285714 0.15714286 0.17142857 0.18571429 0.2 0.21428571 0.22857143 0.24285714 0.25714286 0.27142857 0.28571429 0.3 0.31428571 0.32857143 0.34285714 0.35714286 0.37142857 0.38571429 0.4 0.41428571 0.42857143 0.44285714 0.45714286 0.47142857 0.48571429 0.5 0.51428571 0.52857143 0.54285714 0.55714286 0.57142857 0.58571429 0.6 0.61428571 0.62857143 0.64285714 0.65714286 0.67142857 0.68571429 0.7 0.71428571 0.72857143 0.74285714 0.75714286 0.77142857 0.78571429 0.8 0.81428571 0.82857143 0.84285714 0.85714286 0.87142857 0.88571429 0.9 0.91428571 0.92857143 0.94285714 0.95714286 0.97142857 0.98571429 1 1 1 1 1 1
  arc A30 (343.5341, 45.9448) -> (339.5927, 52.7715) centre (264.6494, 4.9519) ccw
  spline S15 degree 5 poles (339.5927, 52.7715) (339.5342, 52.7754) (339.4174, 52.783) (339.2423, 52.7939) (339.0089, 52.8075) (338.7176, 52.8228) (338.4267, 52.8364) (338.1361, 52.8483) (337.8458, 52.8586) (337.5559, 52.8671) (337.2664, 52.874) (336.9774, 52.8792) (336.6887, 52.8826) (336.4004, 52.8844) (336.1126, 52.8844) (335.8252, 52.8827) (335.5383, 52.8792) (335.2518, 52.874) (334.9658, 52.8671) (334.6803, 52.8583) (334.3953, 52.8478) (334.1108, 52.8356) (333.8269, 52.8215) (333.5435, 52.8056) (333.2607, 52.7879) (332.9784, 52.7684) (332.6967, 52.7471) (332.4156, 52.7239) (332.1352, 52.6989) (331.8553, 52.672) (331.5761, 52.6432) (331.2976, 52.6125) (331.0197, 52.58) (330.7426, 52.5455) (330.4662, 52.509) (330.1905, 52.4707) (329.9155, 52.4303) (329.6413, 52.388) (329.3679, 52.3438) (329.0953, 52.2975) (328.8235, 52.2492) (328.5526, 52.1988) (328.2826, 52.1463) (328.0135, 52.0917) (327.7453, 52.0349) (327.4781, 51.9761) (327.2118, 51.9151) (326.9465, 51.8519) (326.6822, 51.7867) (326.4189, 51.7192) (326.1568, 51.6494) (325.8958, 51.5772) (325.6361, 51.5024) (325.3778, 51.4251) (325.1207, 51.3453) (324.865, 51.263) (324.6103, 51.1784) (324.3569, 51.0917) (324.1046, 51.0026) (323.8538, 50.911) (323.6048, 50.8163) (323.3578, 50.718) (323.1132, 50.6157) (322.871, 50.5095) (322.631, 50.3998) (322.3926, 50.2874) (322.1553, 50.173) (321.9193, 50.0569) (321.6848, 49.9382) (321.4535, 49.815) (321.2274, 49.6841) (321.0524, 49.5707) (320.9251, 49.4797) (320.8422, 49.4162) (320.8012, 49.3838) knots -1 -1 -1 -1 -1 -1 -0.98571429 -0.97142857 -0.95714286 -0.94285714 -0.92857143 -0.91428571 -0.9 -0.88571429 -0.87142857 -0.85714286 -0.84285714 -0.82857143 -0.81428571 -0.8 -0.78571429 -0.77142857 -0.75714286 -0.74285714 -0.72857143 -0.71428571 -0.7 -0.68571429 -0.67142857 -0.65714286 -0.64285714 -0.62857143 -0.61428571 -0.6 -0.58571429 -0.57142857 -0.55714286 -0.54285714 -0.52857143 -0.51428571 -0.5 -0.48571429 -0.47142857 -0.45714286 -0.44285714 -0.42857143 -0.41428571 -0.4 -0.38571429 -0.37142857 -0.35714286 -0.34285714 -0.32857143 -0.31428571 -0.3 -0.28571429 -0.27142857 -0.25714286 -0.24285714 -0.22857143 -0.21428571 -0.2 -0.18571429 -0.17142857 -0.15714286 -0.14285714 -0.12857143 -0.11428571 -0.1 -0.08571429 -0.07142857 -0.05714286 -0.04285714 -0.02857143 -0.01428571 0 0 0 0 0 0
  line L15 (320.8012, 49.3838) -> (314.4257, 44.339)
  arc A31 (311.6562, 44.6176) -> (314.4257, 44.339) centre (313.1847, 45.9074) ccw
  arc A32 (311.6562, 44.6176) -> (304.3151, 51.9586) centre (264.6494, 4.9519) ccw
  arc A33 (304.0366, 54.7282) -> (304.3151, 51.9586) centre (305.6049, 53.4871) ccw
  line L16 (304.0366, 54.7282) -> (309.0814, 61.1036)
  spline S16 degree 5 poles (309.0814, 61.1036) (309.1138, 61.1446) (309.1773, 61.2276) (309.2683, 61.3548) (309.3817, 61.5298) (309.5126, 61.756) (309.6358, 61.9873) (309.7544, 62.2217) (309.8706, 62.4578) (309.985, 62.695) (310.0974, 62.9334) (310.2071, 63.1734) (310.3133, 63.4156) (310.4155, 63.6602) (310.5138, 63.9072) (310.6086, 64.1562) (310.7002, 64.4071) (310.7893, 64.6593) (310.876, 64.9128) (310.9606, 65.1674) (311.0428, 65.4232) (311.1227, 65.6802) (311.2, 65.9386) (311.2747, 66.1982) (311.347, 66.4592) (311.4168, 66.7214) (311.4842, 66.9846) (311.5495, 67.249) (311.6126, 67.5143) (311.6736, 67.7805) (311.7325, 68.0477) (311.7893, 68.3159) (311.8439, 68.585) (311.8964, 68.855) (311.9467, 69.1259) (311.9951, 69.3977) (312.0413, 69.6703) (312.0856, 69.9437) (312.1279, 70.2179) (312.1682, 70.4929) (312.2066, 70.7686) (312.243, 71.045) (312.2775, 71.3222) (312.3101, 71.6) (312.3408, 71.8785) (312.3696, 72.1577) (312.3965, 72.4376) (312.4215, 72.7181) (312.4447, 72.9991) (312.466, 73.2808) (312.4855, 73.5631) (312.5032, 73.8459) (312.5191, 74.1293) (312.5331, 74.4133) (312.5454, 74.6977) (312.5559, 74.9827) (312.5646, 75.2682) (312.5716, 75.5542) (312.5768, 75.8407) (312.5803, 76.1276) (312.582, 76.415) (312.582, 76.7028) (312.5802, 76.9911) (312.5768, 77.2798) (312.5716, 77.5689) (312.5647, 77.8584) (312.5561, 78.1482) (312.5459, 78.4385) (312.534, 78.7291) (312.5203, 79.02) (312.5051, 79.3114) (312.4915, 79.5447) (312.4806, 79.7198) (312.473, 79.8367) (312.4691, 79.8951) knots 0 0 0 0 0 0 0.01428571 0.02857143 0.04285714 0.05714286 0.07142857 0.08571429 0.1 0.11428571 0.12857143 0.14285714 0.15714286 0.17142857 0.18571429 0.2 0.21428571 0.22857143 0.24285714 0.25714286 0.27142857 0.28571429 0.3 0.31428571 0.32857143 0.34285714 0.35714286 0.37142857 0.38571429 0.4 0.41428571 0.42857143 0.44285714 0.45714286 0.47142857 0.48571429 0.5 0.51428571 0.52857143 0.54285714 0.55714286 0.57142857 0.58571429 0.6 0.61428571 0.62857143 0.64285714 0.65714286 0.67142857 0.68571429 0.7 0.71428571 0.72857143 0.74285714 0.75714286 0.77142857 0.78571429 0.8 0.81428571 0.82857143 0.84285714 0.85714286 0.87142857 0.88571429 0.9 0.91428571 0.92857143 0.94285714 0.95714286 0.97142857 0.98571429 1 1 1 1 1 1
  arc A34 (312.4691, 79.8951) -> (305.6424, 83.8365) centre (264.6494, 4.9519) ccw
  spline S17 degree 5 poles (305.6424, 83.8365) (305.5898, 83.8107) (305.4848, 83.7588) (305.3277, 83.6807) (305.1188, 83.5758) (304.8589, 83.4434) (304.6001, 83.3097) (304.3425, 83.1747) (304.086, 83.0385) (303.8307, 82.901) (303.5765, 82.7622) (303.3236, 82.6221) (303.0719, 82.4807) (302.8213, 82.3381) (302.5721, 82.1942) (302.324, 82.049) (302.0773, 81.9026) (301.8318, 81.7548) (301.5876, 81.6058) (301.3447, 81.4555) (301.1032, 81.3039) (300.8629, 81.1511) (300.6241, 80.9969) (300.3866, 80.8415) (300.1505, 80.6847) (299.9158, 80.5267) (299.6825, 80.3674) (299.4507, 80.2068) (299.2203, 80.0449) (298.9914, 79.8816) (298.764, 79.7171) (298.5381, 79.5513) (298.3138, 79.3842) (298.091, 79.2157) (297.8698, 79.046) (297.6502, 78.8749) (297.4323, 78.7025) (297.216, 78.5287) (297.0013, 78.3537) (296.7884, 78.1773) (296.5772, 77.9996) (296.3677, 77.8205) (296.1601, 77.64) (295.9544, 77.4582) (295.7505, 77.2749) (295.5486, 77.0903) (295.3485, 76.9044) (295.1503, 76.7171) (294.954, 76.5284) (294.7597, 76.3383) (294.5676, 76.1468) (294.3777, 75.9538) (294.1902, 75.7592) (294.0051, 75.563) (293.8224, 75.3654) (293.642, 75.1662) (293.4638, 74.9657) (293.2877, 74.7638) (293.1138, 74.5606) (292.9424, 74.3558) (292.774, 74.1493) (292.6093, 73.9406) (292.4486, 73.7298) (292.292, 73.5167) (292.139, 73.3017) (291.9887, 73.0851) (291.8404, 72.8675) (291.6941, 72.6488) (291.5503, 72.4289) (291.4117, 72.2065) (291.2813, 71.9801) (291.1864, 71.7944) (291.1217, 71.6519) (291.0816, 71.5555) (291.0623, 71.5069) knots -1 -1 -1 -1 -1 -1 -0.98571429 -0.97142857 -0.95714286 -0.94285714 -0.92857143 -0.91428571 -0.9 -0.88571429 -0.87142857 -0.85714286 -0.84285714 -0.82857143 -0.81428571 -0.8 -0.78571429 -0.77142857 -0.75714286 -0.74285714 -0.72857143 -0.71428571 -0.7 -0.68571429 -0.67142857 -0.65714286 -0.64285714 -0.62857143 -0.61428571 -0.6 -0.58571429 -0.57142857 -0.55714286 -0.54285714 -0.52857143 -0.51428571 -0.5 -0.48571429 -0.47142857 -0.45714286 -0.44285714 -0.42857143 -0.41428571 -0.4 -0.38571429 -0.37142857 -0.35714286 -0.34285714 -0.32857143 -0.31428571 -0.3 -0.28571429 -0.27142857 -0.25714286 -0.24285714 -0.22857143 -0.21428571 -0.2 -0.18571429 -0.17142857 -0.15714286 -0.14285714 -0.12857143 -0.11428571 -0.1 -0.08571429 -0.07142857 -0.05714286 -0.04285714 -0.02857143 -0.01428571 0 0 0 0 0 0
  line L17 (291.0623, 71.5069) -> (288.0634, 63.9503)
  arc A35 (285.5256, 62.8067) -> (288.0634, 63.9503) centre (286.2045, 64.688) ccw
  arc A36 (285.5256, 62.8067) -> (275.4976, 65.4937) centre (264.6494, 4.9519) ccw
  arc A37 (273.8715, 67.753) -> (275.4976, 65.4937) centre (275.8503, 67.4624) ccw
  line L18 (273.8715, 67.753) -> (275.0527, 75.7967)
  spline S18 degree 5 poles (275.0527, 75.7967) (275.0603, 75.8484) (275.0738, 75.952) (275.089, 76.1077) (275.0997, 76.3159) (275.1, 76.5772) (275.0911, 76.8391) (275.0766, 77.1015) (275.0591, 77.364) (275.0396, 77.6266) (275.0177, 77.8893) (274.9927, 78.1521) (274.9636, 78.4149) (274.9299, 78.6778) (274.8915, 78.9409) (274.849, 79.2039) (274.803, 79.467) (274.754, 79.7299) (274.7024, 79.9928) (274.6483, 80.2556) (274.5916, 80.5182) (274.5323, 80.7808) (274.47, 81.0432) (274.4049, 81.3054) (274.337, 81.5675) (274.2664, 81.8295) (274.1932, 82.0912) (274.1175, 82.3528) (274.0396, 82.6141) (273.9592, 82.8752) (273.8766, 83.136) (273.7917, 83.3966) (273.7044, 83.657) (273.6149, 83.9171) (273.5231, 84.1769) (273.429, 84.4364) (273.3328, 84.6956) (273.2344, 84.9546) (273.134, 85.2132) (273.0314, 85.4715) (272.9268, 85.7294) (272.8201, 85.987) (272.7114, 86.2443) (272.6007, 86.5012) (272.488, 86.7577) (272.3733, 87.0139) (272.2567, 87.2697) (272.1381, 87.5251) (272.0177, 87.7801) (271.8953, 88.0348) (271.7711, 88.289) (271.645, 88.5428) (271.517, 88.7961) (271.3872, 89.0491) (271.2556, 89.3016) (271.1222, 89.5536) (270.987, 89.8052) (270.8501, 90.0564) (270.7113, 90.3071) (270.5709, 90.5573) (270.4287, 90.807) (270.2847, 91.0563) (270.1391, 91.3051) (269.9917, 91.5533) (269.8427, 91.8011) (269.692, 92.0484) (269.5397, 92.2951) (269.3857, 92.5414) (269.23, 92.7871) (269.0728, 93.0322) (268.9139, 93.2769) (268.7855, 93.4722) (268.6884, 93.6184) (268.6234, 93.7158) (268.5908, 93.7644) knots 0 0 0 0 0 0 0.01428571 0.02857143 0.04285714 0.05714286 0.07142857 0.08571429 0.1 0.11428571 0.12857143 0.14285714 0.15714286 0.17142857 0.18571429 0.2 0.21428571 0.22857143 0.24285714 0.25714286 0.27142857 0.28571429 0.3 0.31428571 0.32857143 0.34285714 0.35714286 0.37142857 0.38571429 0.4 0.41428571 0.42857143 0.44285714 0.45714286 0.47142857 0.48571429 0.5 0.51428571 0.52857143 0.54285714 0.55714286 0.57142857 0.58571429 0.6 0.61428571 0.62857143 0.64285714 0.65714286 0.67142857 0.68571429 0.7 0.71428571 0.72857143 0.74285714 0.75714286 0.77142857 0.78571429 0.8 0.81428571 0.82857143 0.84285714 0.85714286 0.87142857 0.88571429 0.9 0.91428571 0.92857143 0.94285714 0.95714286 0.97142857 0.98571429 1 1 1 1 1 1
  arc A38 (268.5908, 93.7644) -> (260.708, 93.7644) centre (264.6494, 4.9519) ccw